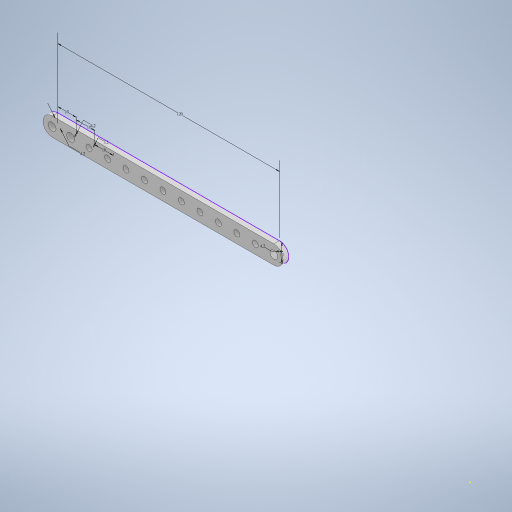
# Autodesk Inventor part: adjustable
Saved by Autodesk Inventor 2023 (Build 270158000, 158)
## iProperties
Created: 2023-04-16
Part Number: adjustable
Material: 一般
Document SubType Name: Modeling
Designer: JOU
Density: 1 g/cm^3
Appearance: 預設
Author: JOU
Autodesk Inventor part; units mm, degrees
ref_plane "YZ Plane" through (0, 0, 0) normal (1, 0, 0) x (0, 1, 0)
ref_plane "XZ Plane" through (0, 0, 0) normal (0, 1, 0) x (-1, 0, 0)
ref_plane "XY Plane" through (0, 0, 0) normal (0, 0, 1) x (1, 0, 0)
sketch "草圖1" plane through (0, 0, 0) normal (0, 0, 1) x (1, 0, 0)
  line L0 (-223.1596, 56.676) -> (-103.1596, 56.676) construction
  line L1 (-223.1596, 51.676) -> (-103.1596, 51.676)
  line L2 (-103.1596, 61.676) -> (-223.1596, 61.676)
  arc A0 (-223.1596, 61.676) -> (-223.1596, 51.676) centre (-223.1596, 56.676) ccw
  arc A1 (-103.1596, 51.676) -> (-103.1596, 61.676) centre (-103.1596, 56.676) ccw
  circle A2 centre (-223.1596, 56.676) radius 2.1
  circle A3 centre (-103.1596, 56.676) radius 2.1
  circle A4 centre (-213.1596, 56.676) radius 2.1
  circle A5 centre (-203.1596, 56.676) radius 1.6
  circle A6 centre (-193.1596, 56.676) radius 1.6
  circle A7 centre (-183.1596, 56.676) radius 1.6
  circle A8 centre (-173.1596, 56.676) radius 1.6
  circle A9 centre (-163.1596, 56.676) radius 1.6
  circle A10 centre (-153.1596, 56.676) radius 1.6
  circle A11 centre (-143.1596, 56.676) radius 1.6
  circle A12 centre (-133.1596, 56.676) radius 1.6
  circle A13 centre (-123.1596, 56.676) radius 1.6
  circle A14 centre (-113.1596, 56.676) radius 1.6
  point P0 (0, 0)
  dimension "d0" = 120
  dimension "d1" = 10
  dimension "d2" = 4.2
  dimension "d3" = 4.2
  dimension "d4" = 4.2
  dimension "d11" = 3.2
  dimension "d12" = 10
  dimension "d13" = 10
  dimension "d16" = 10
  constraints: 15 centre point, 8 end point, 4 point on circle, 4 tangent, 2 coincident, 2 horizontal, 2 point on line, 1 midpoint, 1 parallel, 18 other
  measures "d0" distance of L2.start L2.end
  measures "d1" distance between parallel lines of L1 L2
  measures "d2" diameter of A2
  measures "d3" diameter of A3
  measures "d4" diameter of A4
  measures "d11" diameter of A5
  measures "d12" distance of L0.start A4.centre
  measures "d13" distance of A5.centre A4.centre
  measures "d16" distance of A5.centre A6.centre
extrude "擠出1" add sketch "草圖1" along normal blind 3 contours A0 L2 A1 L1 | A5 | A6 | A7 | A8 | A9 | A10 | A11 | A12 | A13 | A14
extrude "擠出2" cut sketch "草圖1" along normal blind 10 contours A5 | A6 | A7 | A8 | A9 | A10 | A11 | A12 | A13 | A14
